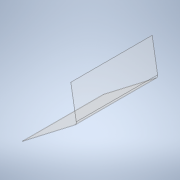
# Autodesk Inventor part: 機体ケツ防護カバー
Saved by Autodesk Inventor 2020.2 (Build 242310000, 310)
## iProperties
Created: 2020-05-27
Part Number: 機体ケツ防護カバー
Material: ポリカーボネート、クリア
Document SubType Name: Modeling
Designer: mozar
Density: 1.2 g/cm^3
Appearance: ポリカーボネート - クリア
Author: mozar
Autodesk Inventor part; units mm, degrees
ref_plane "YZ Plane" through (0, 0, 0) normal (1, 0, 0) x (0, 1, 0)
ref_plane "XZ Plane" through (0, 0, 0) normal (0, 1, 0) x (-1, 0, 0)
ref_plane "XY Plane" through (0, 0, 0) normal (0, 0, 1) x (1, 0, 0)
sketch "スケッチ1" plane through (0, 0, 0) normal (0, 0, 1) x (1, 0, 0)
  line L0 (109.2087, 3) -> (109.2087, 0)
  line L1 (109.2087, -3) -> (109.2087, 0)
  circle A0 centre (111.885, -36) radius 4
  circle A1 centre (47.8869, -85.25) radius 4
  line L2 (109.2087, 3) -> (115.8267, -35.3193)
  line L3 (114.3245, -39.17) -> (50.3264, -88.42)
  line L4 (116.3194, -35.2342) -> (108.7087, 8.833)
  line L5 (108.7087, 8.833) -> (108.7087, 0)
  line L6 (114.6295, -39.5663) -> (50.6314, -88.8163)
  circle A2 centre (111.885, -36) radius 4.5
  line L7 (50.6314, -88.8163) -> (50.3264, -88.42)
  line L8 (109.2087, 3) -> (109.7014, 3.0851)
  point P0 (0, 0)
  dimension "d0" = 0.5
  dimension "d1" = 0.5
  dimension "d2" = 0.5
  constraints: 18 end point, 2 centre point, 2 perpendicular, 2 point on circle, 2 tangent, 2 vertical, 1 parallel, 1 point on line, 7 other
  measures "d0" distance between parallel lines of L2 L4
  measures "d1" distance between parallel lines of L3 L6
  measures "d2" radial gap between concentric circles of A0 A2
extrude "押し出し1" add sketch "スケッチ1" against normal blind 98.8 contours A0 L2 A2 L3 | L2 L8 L4 A2 | A2 L6 L7 L3 picked at (113.4651, -39.9472)
